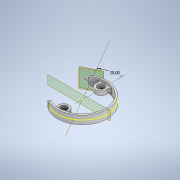
# Autodesk Inventor part: Parachute_Verb
Saved by Autodesk Inventor 2020 (Build 240168000, 168)
## iProperties
Created: 2022-04-20
Part Number: Parachute_Verb
Material: Generisch
Document SubType Name: Modeling
Designer: sp
Density: 1 g/cm^3
Appearance: Vorgabe
Author: sp
## iProperties of the stored document _3D-Druck.ipt
Created: 2022-05-01
Part Number: _3D-Druck
Material: Generisch
Document SubType Name: Modeling
Designer: sp
Density: 1 g/cm^3
Appearance: Vorgabe
Author: sp
Autodesk Inventor part; units mm, degrees
ref_plane "YZ Plane" through (0, 0, 0) normal (1, 0, 0) x (0, 1, 0)
ref_plane "XZ Plane" through (0, 0, 0) normal (0, 1, 0) x (-1, 0, 0)
ref_plane "XY Plane" through (0, 0, 0) normal (0, 0, 1) x (1, 0, 0)
sketch "Skizze1" plane through (0, 0, 0) normal (0, 1, 0) x (-1, 0, 0)
  circle A0 centre (0, 0) radius 28
  circle A1 centre (0, 0) radius 30
  dimension "d0" = 56
  dimension "d1" = 60
  constraints: 2 centre point, 2 coincident
  measures "d0" diameter of A0
  measures "d1" diameter of A1
extrude "Extrusion1" add sketch "Skizze1" along normal mid plane 10
sketch "Skizze2" plane through (0, 0, 0) normal (0, 1, 0) x (-1, 0, 0)
  circle A0 centre (0, 22.5) radius 4.25
  circle A1 centre (0, -22.5) radius 4.25
  line L0 (44.9262, 0) -> (-43.1306, 0) construction
  circle A2 centre (0, -22.5) radius 6.5
  circle A3 centre (0, 22.5) radius 6.5
  line L1 (0, 38.6377) -> (0, -60.2779) construction
  line L2 (3, 29.5) -> (-3, 29.5)
  line L3 (-3, 29.5) -> (-3, -29.5)
  line L4 (-3, -29.5) -> (3, -29.5)
  line L5 (3, -29.5) -> (3, 29.5)
  point P0 (0, 0)
  point P1 (-3, 28.2663)
  point P2 (3, 28.2663)
  point P3 (-3, -28.2663)
  point P4 (3, -28.2663)
  dimension "d4" = 45
  dimension "d5" = 8.5
  dimension "d6" = 8.5
  dimension "d7" = 13
  dimension "d8" = 13
  dimension "d9" = 6
  dimension "d21" = 59
  constraints: 12 end point, 4 centre point, 2 coincident, 2 horizontal, 2 parallel, 2 point on line, 1 perpendicular, 1 symmetric about line, 1 vertical, 2 other
  measures "d4" distance of A1.centre A0.centre
  measures "d5" diameter of A1
  measures "d6" diameter of A0
  measures "d7" diameter of A3
  measures "d8" diameter of A2
  measures "d9" distance between parallel lines of L3 L5
  measures "d21" distance of L2.end L3.end
extrude "Extrusion2" add sketch "Skizze2" along normal mid plane 5 contours A0 L5 A3 | A0 L3 A3 L5 | L5 A3 L3 A0 | A0 L3 A3 | A3 L3 L2 L5 | L5 A1 L3 A2 | A2 L5 A1 | L3 A1 A2 | L3 A1 L5 A2 | A2 L5 L4 L3
sketch "Skizze3" plane through (0, 0, 0) normal (0, 1, 0) x (-1, 0, 0)
  line L0 (-37.328, 53.3099) -> (47.5678, -67.9338) construction
  line L1 (48.5469, 69.3321) -> (-29.5635, -42.2211) construction
  line L2 (0, 56.0595) -> (0, -79.5026) construction
  circle A0 centre (0, 0) radius 30
  circle A1 centre (0, 0) radius 28
  line L3 (19.8236, 28.311) -> (13.732, 19.6114)
  line L4 (14.4871, -20.6897) -> (22.3283, -31.8882)
  point P0 (16.0601, -22.9363)
  point P1 (17.2073, -24.5746)
  point P2 (17.2073, 24.5746)
  point P3 (16.0601, 22.9363)
  dimension "d12" = 110
  dimension "d13" = 35
  dimension "d19" = 56
  dimension "d20" = 60
  constraints: 10 end point, 7 point on line, 3 coincident, 2 centre point, 1 vertical
  measures "d12" angle of L0 L1
  measures "d13" angle of L2 L0
  measures "d19" diameter of A1
  measures "d20" diameter of A0
extrude "Extrusion3" cut sketch "Skizze3" along normal mid plane 10 contours A0 L4 A1 L3 picked at (29.0468, 2.3769)
sketch "Skizze4" plane through (0, 0, 0) normal (0, 1, 0) x (-1, 0, 0)
  line L0 (-8.0451, 13.9345) -> (38.1422, -66.0642) construction
  line L1 (17.2073, -24.5746) -> (16.0601, -22.9363) construction
  line L2 (0, 9.2259) -> (0, -51.7672) construction
  arc A0 (17.2073, 24.5746) -> (17.2073, -24.5746) centre (0, 0) ccw projected
  point P0 (16.6337, -23.7554)
  point P1 (15, -25.9808)
  point P2 (15, -25.9808)
  point P3 (19.2393, -22.9285)
  dimension "d16" = 30
  constraints: 4 end point, 3 point on line, 2 point on circle, 1 vertical, 2 other
  measures "d16" angle of L2 L0
ref_plane "Arbeitsebene3" through (-15.5, 0, -26.8468) normal (-0.4226, 0, -0.9063) x (0, -1, 0)
sketch "Skizze5" plane through (-15.5, 0, -26.8468) normal (-0.4226, 0, -0.9063) x (0, -1, 0)
  point P0 (0, -2.7018)
ref_plane "Arbeitsebene4" through (-15, 0, -25.9808) normal (-0.5, 0, -0.866) x (0, -1, 0)
sketch "Skizze6" plane through (-15, 0, -25.9808) normal (-0.5, 0, -0.866) x (0, -1, 0)
  circle A0 centre (0, 0) radius 2.5131
  point P0 (0, 0)
  constraints: 1 centre point, 1 coincident
extrude "Extrusion5" cut sketch "Skizze6" against normal blind 1
mirror "Spiegeln2" about plane through (0, 0, 0) normal (0, 0, 1) of "Extrusion5"
fillet "Rundung1" radius 4 4 edges at (-16.6337, -5, -23.7554) (-16.6337, 5, -23.7554) (-16.6337, 5, 23.7554) (-16.6337, -5, 23.7554)
fillet "Rundung2" radius 2 4 edges at (3.8552, 0, -27.7333) (-3.8552, 0, -27.7333) (-3.8552, 0, 27.7333) (3.8552, 0, 27.7333)
ref_plane "Arbeitsebene5" through (0, 0, 0) normal (0, 0, 1) x (1, 0, 0)
